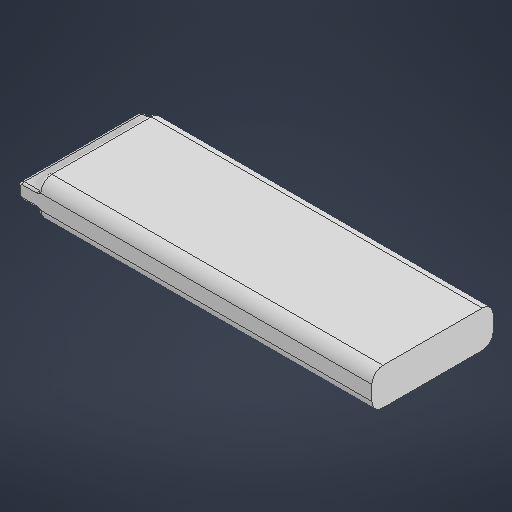
# Autodesk Inventor part: single cell battery
Saved by Autodesk Inventor 2026 (Build 300175050, 175E)
## iProperties
Created: 2025-08-07
Part Number: single cell battery
Material: Generic
Document SubType Name: Modeling
Designer: localuser
Density: 1 g/cm^3
Appearance: Default
Author: localuser
Autodesk Inventor part; units mm, degrees
ref_plane "YZ Plane" through (0, 0, 0) normal (1, 0, 0) x (0, 1, 0)
ref_plane "XZ Plane" through (0, 0, 0) normal (0, 1, 0) x (-1, 0, 0)
ref_plane "XY Plane" through (0, 0, 0) normal (0, 0, 1) x (1, 0, 0)
sketch "Sketch1" plane through (0, 0, 0) normal (0, 1, 0) x (-1, 0, 0)
  line L0 (0, 0) -> (0, -33)
  line L1 (0, -33) -> (96, -33)
  line L2 (96, -33) -> (96, 0)
  line L3 (96, 0) -> (0, 0)
  dimension "d1" = 33
  dimension "d2" = 96
  dimension "d3" = 33
  constraints: 8 end point, 2 perpendicular, 1 vertical
  measures "d1" distance of L0.start L0.end
  measures "d2" distance of L0.end L1.end
  measures "d3" distance of L1.end L2.end
extrude "Extrusion1" add sketch "Sketch1" along normal blind 10
sketch "Sketch2" plane through (0, 10, 0) normal (0, 1, 0) x (1, 0, 0)
  line L0 (-96, 33) -> (-96, 0) projected
  line L1 (-96, 0) -> (-91, 0)
  line L2 (-96, 0) -> (0, 0) projected
  line L3 (-91, 0) -> (-91, 33)
  line L4 (0, 33) -> (-96, 33) projected
  line L5 (-91, 0) -> (-96, 0)
  line L6 (-96, 33) -> (-96, 0)
  line L7 (-96, 33) -> (-91, 33)
  dimension "d6" = 5
  constraints: 10 end point, 2 collinear, 2 perpendicular, 2 point on line
  measures "d6" distance of L0.end L1.end
extrude "Extrusion2" cut sketch "Sketch2" against normal blind 3
sketch "Sketch3" plane through (0, 0, 0) normal (0, -1, 0) x (1, 0, 0)
  line L0 (-96, 0) -> (0, 0) projected
  line L1 (-96, 0) -> (-91, 0)
  line L2 (-91, 0) -> (-91, -33)
  line L3 (-91, -33) -> (-96, -33)
  line L4 (-96, -33) -> (-96, 0)
  dimension "d9" = 5
  dimension "d10" = 33
  constraints: 8 end point, 3 perpendicular, 1 point on line
  measures "d9" distance of L0.start L1.end
  measures "d10" distance of L1.end L2.end
extrude "Extrusion3" cut sketch "Sketch3" against normal blind 3
fillet "Fillet1" radius 3 4 edges at (-45.5, 10, 0) (-45.5, 10, -33) (-45.5, 0, -33) (-45.5, 0, 0)
fillet "Fillet2" radius 1 8 edges at (-91, 0.8787, -32.1213) (-91, 0.8787, -0.8787) (-91, 0, -16.5) (-91, 9.1213, -0.8787) (-91, 9.1213, -32.1213) (-91, 10, -16.5) (-96, 7, -16.5) (-96, 3, -16.5)
fillet "Fillet3" radius 0.5 14 edges at (-93, 7, -33) (-90.5, 7, -33) (-95.7071, 6.7071, -33) (-96, 5, -33) (-95.7071, 3.2929, -33) (-93, 3, -33) (-90.5, 3, -33) (-95.7071, 6.7071, 0) (-96, 5, 0) (-95.7071, 3.2929, 0) (-90.5, 3, 0) (-93, 3, 0) (-90.5, 7, 0) (-93, 7, 0)
body "Solid1"
